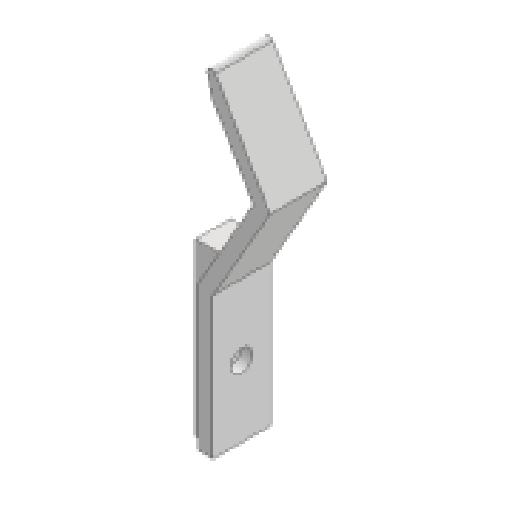
# Autodesk Inventor part: KNUCKLE 3
Saved by Autodesk Inventor 2025.1 (Build 291241020, 241B)
## iProperties
Created: 2024-12-04
Part Number: KNUCKLE 3
Material: Generic
Document SubType Name: Modeling
Designer: ALEXANDERNICHOLS
Density: 1 g/cm^3
Appearance: Default
Author: ALEXANDERNICHOLS
Autodesk Inventor part; units mm, degrees
ref_plane "YZ Plane" through (0, 0, 0) normal (1, 0, 0) x (0, 1, 0)
ref_plane "XZ Plane" through (0, 0, 0) normal (0, 1, 0) x (-1, 0, 0)
ref_plane "XY Plane" through (0, 0, 0) normal (0, 0, 1) x (1, 0, 0)
sketch "Sketch1" plane through (0, 0, 0) normal (0, 0, 1) x (1, 0, 0)
  line L0 (0, 0) -> (0, 50.404)
  line L1 (-5.08, 51.7652) -> (-5.08, 0)
  line L2 (-5.08, 0) -> (0, 0)
  line L3 (-5.08, 51.7652) -> (14.2875, 85.3107)
  line L4 (14.2875, 85.3107) -> (-9.646, 126.7648)
  line L5 (-9.646, 126.7648) -> (-5.2466, 129.3048)
  line L6 (-5.2466, 129.3048) -> (20.1534, 85.3107)
  line L7 (20.1534, 85.3107) -> (0, 50.404)
  line L8 (-5.2466, 129.3048) -> (-0.1666, 110.346)
  dimension "d0" = 51.7652
  dimension "d1" = 5.08
  dimension "d6" = 5.08
  dimension "d7" = 5.08
  dimension "d8" = 30
  dimension "d10" = 120
  dimension "d11" = 50.8
  dimension "d12" = 38.735
  dimension "d13" = 15
  constraints: 18 end point, 3 parallel, 2 perpendicular, 1 point on line, 1 vertical
  measures "d0" distance of L1.start L1.end
  measures "d1" distance between parallel lines of L0 L1
  measures "d6" distance between parallel lines of L7 L3
  measures "d7" distance between parallel lines of L6 L4
  measures "d8" angle of L7 L0
  measures "d10" angle of L1 L5
  measures "d11" distance of L5.end L6.end
  measures "d12" distance of L1.start L3.end
  measures "d13" angle of L4 L8
extrude "Extrusion1" add sketch "Sketch1" along normal blind 20.32 contours L2 L1 L3 L4 L8 L6 L7 L0
fillet "Fillet1" radius 1.5875 1 edges at (-5.2466, 129.3048, 10.16)
sketch "Sketch2" plane through (-5.08, 0, 0) normal (-1, 0, 0) x (0, 0, 1)
  line L0 (0, 0) -> (20.32, 0) projected
  line L1 (3.937, 0) -> (16.383, 0)
  line L2 (16.383, 0) -> (16.383, 60.5536)
  line L3 (16.383, 60.5536) -> (3.937, 60.5536)
  line L4 (3.937, 60.5536) -> (3.937, 0)
  point P0 (10.16, 0)
  point P1 (16.383, 0)
  dimension "d15" = 12.446
  dimension "d16" = 6.223
  dimension "d17" = 60.5536
  constraints: 8 end point, 2 parallel, 1 horizontal, 1 midpoint, 1 perpendicular, 1 point on line
  measures "d15" distance between parallel lines of L4 L2
  measures "d16" distance from line of point (10.16, 0) L2
  measures "d17" distance of L3.end L1.start
extrude "Extrusion2" add sketch "Sketch2" along normal blind 5.08
sketch "Sketch3" plane through (0, 0, 0) normal (1, 0, 0) x (0, 0, -1)
  circle A0 centre (-10.16, 25.202) radius 1.778
  line L0 (0, 0) -> (0, 50.404) projected
  line L1 (0, 0) -> (-20.32, 0) projected
  point P0 (0, 25.202)
  point P1 (-10.16, 0)
  dimension "d20" = 3.556
  constraints: 2 midpoint, 1 centre point, 1 horizontal alignment, 1 vertical alignment
  measures "d20" diameter of A0
extrude "Extrusion3" cut sketch "Sketch3" against normal blind 18.7325
sketch "Sketch4" plane through (0, 0, 0) normal (1, 0, 0) x (0, 0, -1)
  circle A0 centre (-10.16, 25.202) radius 1.778 projected
  line L0 (0, 0) -> (0, 50.404) projected
  line L1 (0, 50.404) -> (-20.32, 50.404) projected
  line L2 (-20.32, 0) -> (-20.32, 50.404) projected
  line L3 (0, 0) -> (-20.32, 0) projected
  circle A1 centre (-10.16, 25.202) radius 3.81
  dimension "d23" = 7.62
  constraints: 1 centre point, 1 coincident
  measures "d23" diameter of A1
extrude "Extrusion4" cut sketch "Sketch4" against normal blind 4.0132 contours A1
sketch "Sketch5" plane through (-5.08, 0, 0) normal (1, 0, 0) x (0, 0, -1)
  line L0 (-3.937, 51.7652) -> (-16.383, 51.7652) projected
  line L1 (-3.937, 60.5536) -> (-3.937, 51.7652) projected
  line L2 (-16.383, 60.5536) -> (-3.937, 60.5536) projected
  line L3 (-16.383, 51.7652) -> (-16.383, 60.5536) projected
  point P0 (0, 0)
extrude "Extrusion5" add sketch "Sketch5" against normal up to surface surface through (14.2875, 85.3107, 0) normal (-0.8660254, 0.5, 0)
equation "\"d16\" = 0.5 * d15"
body "Solid1"
